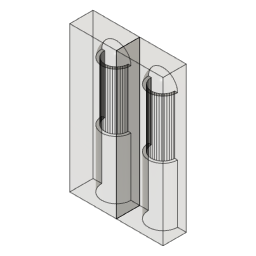
Mót fyrir plast v9 (Autodesk Fusion 360 design; units mm, degrees)
Autodesk Fusion 360 part; units mm, degrees
note: some values were not read from the file. Chosen so that the rebuilt part matches the saved one: which bodies a step acts on.
sketch "Sketch1" plane through (0, 0, 0) normal (0, 0, 1) x (1, 0, 0)
  circle A0 centre (50, 25) radius 5
  dimension "d1" = 10
  measures "d1" diameter of A0
extrude "Extrude1" add sketch "Sketch1" along normal blind 40 makes body 1
sphere "SpherePrimitive1" add diameter 10 placed x (-1, 0, 0) y (0, -1, 0) z (0, 0, 1) at (50, 25, 40) bodies 1
sketch "Sketch4" plane through (0, 0, 0) normal (0, 1, 0) x (1, 0, 0)
sketch "Sketch5" plane through (0, 0, 0) normal (0, 0, -1) x (1, 0, 0)
  circle A0 centre (50, -25) radius 5
  circle A1 centre (50, -25) radius 4
  dimension "d7" = 8
  constraint concentric A0 A1
  measures "d7" diameter of A1
extrude "Extrude3" add sketch "Sketch5" against normal blind 40 separate body contours A1 makes body 2
sketch "Sketch9" plane through (0, 0, 0) normal (0, 1, 0) x (1, 0, 0)
  line L0 (45, -20) -> (55, -20)
  line L1 (55, -20) -> (55, -40)
  line L2 (55, -40) -> (45, -40)
  line L3 (45, -40) -> (45, -20)
  constraint horizontal L0
  constraint vertical L1
  constraint horizontal L2
  constraint vertical L3
extrude "Extrude4" cut sketch "Sketch9" along normal blind 21 bodies 1
pattern_circular "C-Pattern1" count 40 over 360 about axis through (50, 25, 0) along (0, 0, 1) of "Extrude4"
sketch "Sketch10" plane through (0, 0, 0) normal (0, 0, -1) x (1, 0, 0)
  circle A0 centre (50, -25) radius 4
  line L0 (58, -17) -> (42, -17)
  line L1 (42, -17) -> (42, -33)
  line L2 (42, -33) -> (58, -33)
  line L3 (58, -33) -> (58, -17)
  line L4 (58, -17) -> (42, -33) construction
  line L5 (42, -17) -> (58, -33) construction
  point P0 (50, -25)
  constraint horizontal L0
  constraint perpendicular L0 L1
  constraint parallel L0 L2
  constraint parallel L1 L3
  constraint coincident L4 P0
  constraint coincident L5 P0
  constraint coincident P0 A0.centre
extrude "Extrude5" add sketch "Sketch10" along normal blind 0 and the other way blind 50 separate body contours A0 | L0 L1 L2 L3 makes body 3
sketch "Sketch11" plane through (42, 0, 0) normal (-1, 0, 0) x (0, -1, 0)
  line L0 (-33, 50) -> (-33, 0)
  line L1 (-33, 0) -> (-17, 0)
  line L2 (-17, 0) -> (-17, 50)
  line L3 (-17, 50) -> (-33, 50)
  line L4 (-25, 50) -> (-25, 0)
  constraint midpoint L3 L4.start
  constraint midpoint L1 L4.end
split "Split1" by curves path "Sketch11" along L4 bodies 3 makes body 4 at (47.3333, 33, 16.6667)
combine "Combine1" operation cut target body 3 tool bodies 1 2 keep tools result as body 5 in component "Component'"
combine "Combine1'" operation cut target body 4 tool bodies 2 1 keep tools result as body 6 in component "Component''"
move_body "Move1" bodies 6 to x (1, 0, 0) y (0, 1, 0) z (0, 0, 1) at (-25, -8, 0) in component "Component''"
move_body "Move2" bodies 6 to x (-1, 0, 0) y (0, -1, 0) z (0, 0, 1) at (34, 50, 0) in component "Component''"
move_body "Move3" bodies 6 to x (1, 0, 0) y (0, 1, 0) z (0, 0, 1) at (21, -8, 0) in component "Component''"
move_body "Move4" bodies 6 to x (1, 0, 0) y (0, 1, 0) z (0, 0, 1) at (4, 0, 0) in component "Component''"
sketch "Sketch12" plane through (0, 0, 0) normal (0, 1, 0) x (1, 0, 0)
  line L0 (69, -58) -> (14, -58)
  line L1 (14, -58) -> (14, 13)
  line L2 (14, 13) -> (69, 13)
  line L3 (69, 13) -> (69, -58)
  constraint horizontal L0
  constraint vertical L1
  constraint horizontal L2
  constraint vertical L3
extrude "Extrude6" add sketch "Sketch12" along normal blind 30 from surface at 17 separate body makes body 7
sketch "Sketch13" plane through (0, 17, 0) normal (0, -1, 0) x (1, 0, 0)
  line L0 (26, 50) -> (26, 0)
  line L1 (26, 0) -> (42, 0)
  line L2 (42, 0) -> (42, 50)
  line L3 (42, 50) -> (26, 50)
  line L4 (66, 58) -> (18, 58)
  line L5 (18, 58) -> (18, -13)
  line L6 (18, -13) -> (66, -13)
  line L7 (66, -13) -> (66, 58)
  line L8 (8, -23) -> (76, -23)
  line L9 (76, -23) -> (76, 68)
  line L10 (76, 68) -> (8, 68)
  line L11 (8, 68) -> (8, -23)
  dimension "d30" = 10
  constraint horizontal L4
  constraint vertical L5
  constraint horizontal L6
  constraint vertical L7
extrude "Extrude7" add sketch "Sketch13" against normal blind 30 separate body contours L8 L9 L10 L11 makes body 8
sketch "Sketch14" plane through (0, 17, 0) normal (0, -1, 0) x (1, 0, 0)
  line L0 (42, 50) -> (42, 0)
  line L1 (42, 0) -> (58, 0)
  line L2 (58, 0) -> (58, 50)
  line L3 (58, 50) -> (42, 50)
  line L4 (69, 26) -> (14, 26)
  line L5 (14, 26) -> (14, 22.5)
  line L6 (14, 22.5) -> (69, 22.5)
  line L7 (69, 22.5) -> (69, 26)
  constraint horizontal L4
  constraint vertical L5
  constraint horizontal L6
  constraint vertical L7
extrude "Extrude8" add sketch "Sketch14" against normal blind 2 separate body contours L0 L2 L4 L6 | L0 L4 L5 L6 | L2 L4 L6 L7 makes body 9
component "Component'" placed x (1, 0, 0) y (0, 1, 0) z (0, 0, 1) at (0, 0, 0)
component "Component''" placed x (1, 0, 0) y (0, 1, 0) z (0, 0, 1) at (0, 0, 0)
hidden bodies 1 2 3 4 7 8 9
named bodies: "Stock"
